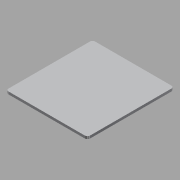
# Autodesk Inventor part: Base plate
Saved by Autodesk Inventor 2017 (Build 210142000, 142)
## iProperties
Created: 2016-12-06
Part Number: Base plate
Material: Aluminum 6061
Document SubType Name: Modeling
Designer: qupec
Density: 2.7 g/cm^3
Appearance: Aluminum - Flat
Author: qupec
Autodesk Inventor part; units mm, degrees
ref_plane "YZ Plane" through (0, 0, 0) normal (1, 0, 0) x (0, 1, 0)
ref_plane "XZ Plane" through (0, 0, 0) normal (0, 1, 0) x (-1, 0, 0)
ref_plane "XY Plane" through (0, 0, 0) normal (0, 0, 1) x (1, 0, 0)
sketch "Sketch1" plane through (0, 0, 0) normal (0, 1, 0) x (-1, 0, 0)
  line L0 (50.8, 53.975) -> (-50.8, 53.975)
  line L1 (-50.8, 53.975) -> (-50.8, -53.975)
  line L2 (-50.8, -53.975) -> (50.8, -53.975)
  line L3 (50.8, -53.975) -> (50.8, 53.975)
  point P0 (0, 0)
  dimension "d0" = 107.95
  dimension "d1" = 101.6
  dimension "d2" = 50.8
  dimension "d3" = 53.975
  constraints: 8 end point, 2 parallel, 1 horizontal, 1 perpendicular
  measures "d0" distance of L2.end L0.start
  measures "d1" distance of L0.start L0.end
  measures "d2" distance from line of point (0, 0) L1
  measures "d3" distance from line of point (0, 0) L0
extrude "Extrusion1" add sketch "Sketch1" along normal blind 3.175
sketch "Sketch4" plane through (0, 3.175, 0) normal (0, 1, 0) x (1, 0, 0)
  circle A0 centre (44.45, 47.625) radius 3.175
  circle A1 centre (44.45, -47.625) radius 3.175
  circle A2 centre (-41.91, -29.845) radius 3.175
  line L0 (50.8, 53.975) -> (-50.8, 53.975) projected
  line L1 (50.8, -53.975) -> (50.8, 53.975) projected
  line L2 (-50.8, -53.975) -> (50.8, -53.975) projected
  line L3 (-50.8, 53.975) -> (-50.8, -53.975) projected
  circle A3 centre (-41.91, 29.845) radius 3.175
  point P0 (0, 0)
  dimension "d20" = 6.35
  dimension "d21" = 6.35
  dimension "d22" = 6.35
  dimension "d23" = 6.35
  dimension "d24" = 6.35
  dimension "d25" = 6.35
  dimension "d26" = 6.35
  dimension "d27" = 24.13
  dimension "d28" = 8.89
  dimension "d32" = 6.35
  dimension "d33" = 24.13
  dimension "d34" = 8.89
  constraints: 4 centre point
  measures "d20" diameter of A2
  measures "d21" diameter of A1
  measures "d22" diameter of A0
  measures "d23" distance from line of L0 A0.centre
  measures "d24" distance from line of L1 A0.centre
  measures "d25" distance from line of L1 A1.centre
  measures "d26" distance from line of L2 A1.centre
  measures "d27" distance from line of L2 A2.centre
  measures "d28" distance from line of L3 A2.centre
  measures "d32" diameter of A3
  measures "d33" distance from line of L0 A3.centre
  measures "d34" distance from line of L3 A3.centre
extrude "Extrusion6" [suppressed]
fillet "Fillet1" radius 3.175 4 edges at (-50.8, 1.5875, 53.975) (50.8, 1.5875, 53.975) (50.8, 1.5875, -53.975) (-50.8, 1.5875, -53.975)
sketch "Sketch6" plane through (0, 0, 0) normal (0, -1, 0) x (1, 0, 0)
  circle A0 centre (-33.4435, 47.625) radius 1.4224 projected
  circle A1 centre (-26.7125, 40.894) radius 1.4224 projected
  line L0 (-26.7125, -40.3479) -> (-12.425, -40.3479)
  circle A2 centre (-19.9815, 47.625) radius 1.4224 projected
  circle A3 centre (-35.08, 13.8268) radius 1.4224 projected
  circle A4 centre (-26.06, 13.8268) radius 1.4224 projected
  circle A5 centre (-35.08, -14.1576) radius 1.4224 projected
  circle A6 centre (-26.06, -14.1576) radius 1.4224 projected
  circle A7 centre (-33.4435, -47.625) radius 1.4224 projected
  circle A8 centre (-26.7125, -40.894) radius 1.4224 projected
  circle A9 centre (-19.9815, -47.625) radius 1.4224 projected
  point P0 (0, 0)
  constraints: 2 end point, 1 horizontal, 2 other
extrude "Extrusion7" cut sketch "Sketch6" against normal through all
equation "\"d2\" = 0.5 * d1"
equation "\"d3\" = 0.5 * d0"
equation "\"d21\" = d20"
equation "\"d22\" = d20"
equation "\"d24\" = d23"
equation "\"d25\" = d24"
equation "\"d26\" = d23"
equation "\"d32\" = d20"
equation "\"d33\" = d27"
equation "\"d34\" = d28"
body "Solid1"
